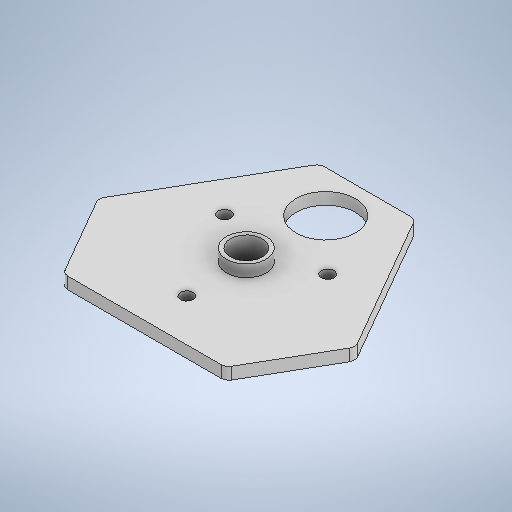
# Autodesk Inventor part: Draw_Pen
Saved by Autodesk Inventor 2025 (Build 290162000, 162)
## iProperties
Created: 2026-06-13
Part Number: Draw_Pen
Material: Generic
Document SubType Name: Sheet Metal
Designer: MSI
Density: 1 g/cm^3
Sheet Metal Rule: Default_mm
Appearance: Default
Author: MSI
Autodesk Inventor part; units mm, degrees
ref_plane "YZ Plane" through (0, 0, 0) normal (1, 0, 0) x (0, 1, 0)
ref_plane "XZ Plane" through (0, 0, 0) normal (0, 1, 0) x (-1, 0, 0)
ref_plane "XY Plane" through (0, 0, 0) normal (0, 0, 1) x (1, 0, 0)
sketch "Sketch1" plane through (0, 0, 0) normal (0, 1, 0) x (-1, 0, 0)
  circle A0 centre (-12.9904, -7.5) radius 1.6
  circle A1 centre (12.9904, -7.5) radius 1.6
  circle A2 centre (0, 15) radius 1.6
  line L0 (31.4449, 6.6077) -> (21.0222, 24.6603)
  line L1 (10.8453, -30.5359) -> (-10.8453, -30.5359)
  line L2 (-21.0222, 24.6603) -> (-31.8675, 5.8756)
  line L3 (-31.8675, 3.8756) -> (-12.5774, -29.5359)
  line L4 (-19.2902, 25.6603) -> (19.2902, 25.6603)
  line L5 (20.4449, 25.6603) -> (31.8675, 5.8756)
  line L6 (31.8675, 3.8756) -> (12.5774, -29.5359)
  arc A3 (21.0222, 24.6603) -> (19.2902, 25.6603) centre (19.2902, 23.6603) ccw
  arc A4 (31.8675, 3.8756) -> (31.8675, 5.8756) centre (30.1355, 4.8756) ccw
  arc A5 (10.8453, -30.5359) -> (12.5774, -29.5359) centre (10.8453, -28.5359) ccw
  arc A6 (-12.5774, -29.5359) -> (-10.8453, -30.5359) centre (-10.8453, -28.5359) ccw
  arc A7 (-19.2902, 25.6603) -> (-21.0222, 24.6603) centre (-19.2902, 23.6603) ccw
  arc A8 (-31.8675, 5.8756) -> (-31.8675, 3.8756) centre (-30.1355, 4.8756) ccw
  circle A9 centre (0, 0) radius 4
  circle A10 centre (0, 0) radius 5
  dimension "d41" = 360
  dimension "d76" = 2
  dimension "d84" = 8
  dimension "d86" = 10
  constraints: 14 end point, 12 point on circle, 12 tangent, 11 centre point, 5 equal radius, 2 coincident, 2 horizontal, 1 point on line, 7 other
  measures "d76" radius of A3
  measures "d84" diameter of A9
  measures "d86" diameter of A10
extrude "Extrusion8" add sketch "Sketch1" along normal blind 3 contours L5 A4 L6 A5 L1 A6 L3 A8 L2 A7 L4 A3 L0
extrude "Extrusion9" add sketch "Sketch1" along normal blind 6 contours A10
sketch "Sketch4" plane through (0, 3, 0) normal (0, 1, 0) x (1, 0, 0)
  point P0 (0, 0)
sketch "Sketch5" plane through (0, 3, 0) normal (0, 1, 0) x (1, 0, 0)
  circle A0 centre (0, 20) radius 7.5
  point P0 (0, 0)
  dimension "d91" = 15
  constraints: 1 centre point
  measures "d91" diameter of A0
extrude "Extrusion10" cut sketch "Sketch5" against normal blind 6
equation "\"BendRadius\" = Thickness"
equation "\"BendReliefWidth\" = Thickness"
equation "\"BendReliefDepth\" = 0.5 * Thickness"
equation "\"CornerReliefSize\" = 4 * Thickness"
equation "\"MinimumRemnant\" = 2 * Thickness"
equation "\"TransitionRadius\" = BendRadius"
equation "\"JacobiRadiusSize\" = BendRadius"
equation "\"GapSize\" = Thickness"
equation "\"Thickness\" = 0.5"
body "Solid3"
